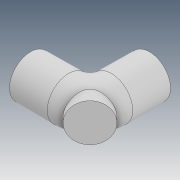
# Autodesk Inventor part: MtoM90degree
Saved by Autodesk Inventor 2020 (Build 240168000, 168)
## iProperties
Created: 2020-05-04
Part Number: MtoM90degree
Material: Generic
Document SubType Name: Modeling
Designer: Theo Cominotto
Density: 1 g/cm^3
Appearance: Default
TMStart: 22,000 mm
TMEnd: 22,400 mm
WallT: 1,600 mm
TDepth: 20,000 mm
BendR: 11,200 mm
Author: Theo Cominotto
Autodesk Inventor part; units mm, degrees
ref_plane "XZ Plane" through (0, 0, 0) normal (0, 1, 0) x (-1, 0, 0)
ref_plane "XY Plane" through (0, 0, 0) normal (0, 0, 1) x (1, 0, 0)
sketch "Sketch1" plane through (0, 0, 0) normal (0, 0, 1) x (1, 0, 0)
  line L0 (0, 0) -> (0, 11) construction
  line L1 (0, 0) -> (20, 0) construction
  line L2 (20, 0) -> (20, 11.2) construction
  line L3 (0, 11) -> (20, 11.2)
  line L4 (0, 9.4) -> (20, 9.4)
  line L5 (20, 9.4) -> (20, 11.2)
  line L6 (0, 9.4) -> (0, 11)
  dimension "d0" = 11
  dimension "d1" = 20
  dimension "d2" = 11.2
  dimension "d3" = 1.6
  constraints: 14 end point, 2 collinear, 2 perpendicular, 2 point on line, 1 horizontal, 1 vertical
  measures "d0" distance of L0.start L0.end
  measures "d1" distance of L0.start L1.end
  measures "d2" distance of L1.end L2.end
  measures "d3" distance of L0.end L4.start
sketch "Sketch1 outline for Revolution1" plane through (0, 0, 0) normal (0, 0, 1) x (1, 0, 0)
  line L0 (20, 9.4) -> (20, 11.2)
  line L1 (0, 9.4) -> (20, 9.4)
  line L2 (0, 11) -> (0, 9.4)
  line L3 (20, 11.2) -> (0, 11)
revolve "Revolution1" add sketch "Sketch1 outline for Revolution1" angle 360 about axis through (0, 0, 0) along (1, 0, 0)
sketch "Sketch2" plane through (20, 0, 0) normal (1, 0, 0) x (0, 0, -1)
  line L0 (0, 0) -> (11.2, 0) construction
  circle A0 centre (0, 0) radius 11.2 construction
  line L1 (11.2, 0) -> (11.2, 11.2) construction
  circle A1 centre (0, 0) radius 11.2
  circle A2 centre (0, 0) radius 9.4 projected
  dimension "d5" = 11.2
  constraints: 4 end point, 1 centre point, 1 coincident, 1 horizontal, 1 horizontal alignment, 1 vertical, 1 other
  measures "d5" distance of L0.start L0.end
sketch "Sketch2 outline for Revolution2" plane through (20, 0, 0) normal (1, 0, 0) x (0, 0, -1)
  circle A0 centre (0, 0) radius 11.2
  circle A1 centre (0, 0) radius 9.4
revolve "Revolution2" add sketch "Sketch2 outline for Revolution2" angle 90 about axis through (20, 0, -11.2) along (0, 1, 0)
sketch "Sketch3" plane through (0, 0, 0) normal (0, 1, 0) x (-1, 0, 0)
  line L0 (-42.4, -11.2) -> (-20, -11.2) construction
  line L1 (-31.2, -11.2) -> (-31.2, -31.2) construction
  line L2 (-31.2, -11.2) -> (-11.2, -11.2) construction
  line L3 (-31.2, -31.2) -> (-20.2, -31.2) construction
  line L4 (-20.2, -31.2) -> (-20, -11.2)
  line L5 (-20.2, -31.2) -> (-21.8, -31.2)
  line L6 (-21.8, -31.2) -> (-21.8, -11.2)
  line L7 (-20, -11.2) -> (-21.8, -11.2)
  point P0 (0, 0)
  dimension "d7" = 20
  dimension "d8" = 90
  dimension "d9" = 11
  dimension "d10" = 1.6
  constraints: 14 end point, 4 perpendicular, 2 point on line, 1 collinear, 1 horizontal, 1 midpoint
  measures "d7" distance of L1.start L1.end
  measures "d8" angle of L1 L2
  measures "d9" distance of L1.end L3.end
  measures "d10" distance of L3.end L5.end
sketch "Sketch3 outline for Revolution3" plane through (0, 0, 0) normal (0, 1, 0) x (-1, 0, 0)
  line L0 (-20.2, -31.2) -> (-20, -11.2)
  line L1 (-21.8, -31.2) -> (-20.2, -31.2)
  line L2 (-21.8, -11.2) -> (-21.8, -31.2)
  line L3 (-20, -11.2) -> (-21.8, -11.2)
revolve "Revolution3" add sketch "Sketch3 outline for Revolution3" angle 360 about axis through (31.2, 0, -11.2) along (0, 0, -1)
ref_plane "Work Plane2" through (21.213203, 0, 21.213203) normal (0.7071068, 0, 0.7071068) x (0, 1, 0)
ref_plane "Work Plane1" through (0, 0, 0) normal (0.7071068, 0, 0.7071068) x (0, 1, 0)
sketch "Sketch4" plane through (21.213203, 0, 21.213203) normal (0.7071068, 0, 0.7071068) x (0, 1, 0)
  ellipse E0 centre (0, -14.142136) end of major axis (11.2, -14.142136) minor radius 7.919596 construction
  ellipse E1 centre (0, -29.981328) end of major axis (11.2, -29.981328) minor radius 7.919596 construction
  line L0 (0, -14.142136) -> (0, -29.981328) construction
  circle A0 centre (0, -22.061732) radius 10
  point P0 (0, 0)
  dimension "d14" = 20
  constraints: 2 end point, 2 vertical alignment, 1 centre point, 1 coincident, 1 vertical
  measures "d14" diameter of A0
sketch "Sketch4 outline for Extrusion1" plane through (21.213203, 0, 21.213203) normal (0.7071068, 0, 0.7071068) x (0, 1, 0)
  circle A0 centre (0, -22.061732) radius 10
extrude "Extrusion1" add sketch "Sketch4 outline for Extrusion1" against normal up to surface
equation "\"d0\" = 0.5 * TMStart"
equation "\"d1\" = TDepth"
equation "\"d2\" = 0.5 * TMEnd"
equation "\"d3\" = WallT"
equation "\"d5\" = BendR"
equation "\"d7\" = TDepth"
equation "\"d9\" = 0.5 * TMStart"
equation "\"d10\" = WallT"
equation "\"TMStart\" = 22"
equation "\"TMEnd\" = 22.4"
equation "\"WallT\" = 1.6"
equation "\"TDepth\" = 20"
equation "\"BendR\" = 0.5 * TMEnd"
body "Solid1"
